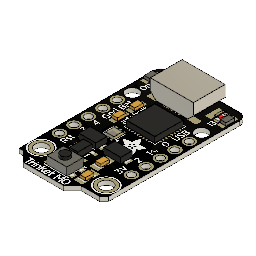
3500 Trinket M0 (Autodesk Fusion 360 design; units mm, degrees)
Autodesk Fusion 360 part; units mm, degrees
sketch "pcb" plane through (0, 0, 0) normal (0, 0, 1) x (1, 0, 0)
  arc A0 (7.62, 11.43) -> (6.35, 12.7) centre (6.35, 11.43) ccw
  line L0 (-6.858, -12.192) -> (-7.62, -12.192)
  line L1 (-7.62, -12.192) -> (-7.62, 11.43)
  line L2 (2.413, 12.319) -> (2.794, 12.7)
  line L3 (7.62, -11.684) -> (6.858, -12.446)
  line L4 (6.858, -12.446) -> (3.556, -12.446)
  line L5 (2.032, -13.97) -> (-5.08, -13.97)
  line L6 (3.556, -12.446) -> (2.032, -13.97)
  line L7 (-2.794, 12.7) -> (-2.413, 12.319)
  circle A1 centre (6.096, 6.223) radius 1.1
  line L8 (2.794, 12.7) -> (6.35, 12.7)
  arc A2 (-6.35, 12.7) -> (-7.62, 11.43) centre (-6.35, 11.43) ccw
  line L9 (-6.35, 12.7) -> (-2.794, 12.7)
  circle A3 centre (-6.096, 6.223) radius 1.1
  line L10 (-2.413, 12.319) -> (2.413, 12.319)
  line L11 (7.62, 11.43) -> (7.62, -11.684)
  line L12 (-5.08, -13.97) -> (-6.858, -12.192)
  circle A4 centre (-6.3246, 3.81) radius 0.635
  circle A5 centre (6.35, 3.81) radius 0.635
  circle A6 centre (6.35, 1.27) radius 0.635
  circle A7 centre (6.35, -1.27) radius 0.635
  circle A8 centre (6.35, -3.81) radius 0.635
  circle A9 centre (6.35, -6.35) radius 0.635
  circle A10 centre (-6.3246, 1.27) radius 0.635
  circle A11 centre (-6.3246, -1.27) radius 0.635
  circle A12 centre (-6.3246, -3.81) radius 0.635
  circle A13 centre (-6.3246, -6.35) radius 0.635
  circle A14 centre (-5.715, -10.16) radius 1.1
  circle A15 centre (5.715, -10.16) radius 1.1
  dimension "d1" = 1.27
  dimension "d2" = 1.27
  dimension "d5" = 0
  dimension "d6" = -2.54
  dimension "d9" = 0
  dimension "d10" = -2.54
  dimension "d11" = 2.2
  dimension "d12" = 2.2
  dimension "d13" = 2.2
  dimension "d14" = 2.2
  measures "d1" diameter of A4
  measures "d2" diameter of A5
  measures "d11" diameter of A14
  measures "d12" diameter of A15
  measures "d13" diameter of A1
  measures "d14" diameter of A3
extrude "Extrude1" add sketch "pcb" along normal blind 0.8 makes body 1
sketch "usb" plane through (0, 0, 0.8) normal (0, 0, 1) x (-1, 0, 0)
  circle A0 centre (-6.35, -3.81) radius 0.635
  circle A1 centre (-6.35, 6.35) radius 0.635
  circle A2 centre (5.715, 10.16) radius 1.1
  circle A3 centre (6.3246, -3.81) radius 0.635
  circle A4 centre (6.3246, 6.35) radius 0.635
  circle A5 centre (-6.096, -6.223) radius 1.1
  circle A6 centre (-6.35, -1.27) radius 0.635
  circle A7 centre (6.3246, -1.27) radius 0.635
  circle A8 centre (6.096, -6.223) radius 1.1
  circle A9 centre (6.3246, 1.27) radius 0.635
  circle A10 centre (-5.715, 10.16) radius 1.1
  circle A11 centre (-6.35, 1.27) radius 0.635
  circle A12 centre (-6.35, 3.81) radius 0.635
  circle A13 centre (6.3246, 3.81) radius 0.635
  arc A14 (-7.62, -11.43) -> (-6.35, -12.7) centre (-6.35, -11.43) ccw
  line L0 (-6.35, -12.7) -> (-2.794, -12.7)
  line L1 (-2.794, -12.7) -> (-2.413, -12.319)
  line L2 (-2.413, -12.319) -> (2.413, -12.319)
  line L3 (2.413, -12.319) -> (2.794, -12.7)
  line L4 (2.794, -12.7) -> (6.35, -12.7)
  arc A15 (6.35, -12.7) -> (7.62, -11.43) centre (6.35, -11.43) ccw
  line L5 (7.62, -11.43) -> (7.62, 12.192)
  line L6 (7.62, 12.192) -> (6.858, 12.192)
  line L7 (6.858, 12.192) -> (5.08, 13.97)
  line L8 (5.08, 13.97) -> (-2.032, 13.97)
  line L9 (-2.032, 13.97) -> (-3.556, 12.446)
  line L10 (-3.556, 12.446) -> (-6.858, 12.446)
  line L11 (-6.858, 12.446) -> (-7.62, 11.684)
  line L12 (-7.62, 11.684) -> (-7.62, -11.43)
  line L13 (3.8, -12.7) -> (-3.8, -12.7)
  line L14 (-3.8, -12.7) -> (-3.8, -7.1)
  line L15 (-3.8, -7.1) -> (3.8, -7.1)
  line L16 (3.8, -7.1) -> (3.8, -12.7)
  line L17 (3.8, -12.7) -> (-3.8, -7.1) construction
  line L18 (-3.8, -12.7) -> (3.8, -7.1) construction
  line L19 (0, -9.9) -> (0, 0) construction
  point P0 (0, -9.9)
  dimension "d17" = 7.6
  dimension "d18" = 5.6
  dimension "d19" = 9.9
  measures "d17" distance of L14.end L15.end
  measures "d18" distance of L13.end L14.end
  measures "d19" distance of L19.end L19.start
extrude "Extrude2" add sketch "usb" along normal blind 3 separate body contours L0 L1 L2 L3 L4 L13 L14 L15 L16 | L1 L2 L3 L13 makes body 2
chamfer "Chamfer1" distance 1 angle 45 2 edges at (3.8, 9.9, 0.8) (-3.8, 9.9, 0.8) on bodies 2
shell "Shell1" thickness 0.4 removed faces 1 at (-0.9333, 12.7, 2.8) on bodies 2
sketch "samd21" plane through (0, 0, 0.8) normal (0, 0, 1) x (-1, 0, 0)
  circle A0 centre (-6.35, -3.81) radius 0.635
  circle A1 centre (-6.35, 6.35) radius 0.635
  circle A2 centre (5.715, 10.16) radius 1.1
  circle A3 centre (6.3246, -3.81) radius 0.635
  circle A4 centre (6.3246, 6.35) radius 0.635
  circle A5 centre (-6.096, -6.223) radius 1.1
  circle A6 centre (-6.35, -1.27) radius 0.635
  circle A7 centre (6.3246, -1.27) radius 0.635
  circle A8 centre (6.096, -6.223) radius 1.1
  circle A9 centre (6.3246, 1.27) radius 0.635
  circle A10 centre (-5.715, 10.16) radius 1.1
  circle A11 centre (-6.35, 1.27) radius 0.635
  circle A12 centre (-6.35, 3.81) radius 0.635
  circle A13 centre (6.3246, 3.81) radius 0.635
  arc A14 (-7.62, -11.43) -> (-6.35, -12.7) centre (-6.35, -11.43) ccw
  line L0 (-6.35, -12.7) -> (-2.794, -12.7)
  line L1 (-2.794, -12.7) -> (-2.413, -12.319)
  line L2 (-2.413, -12.319) -> (2.413, -12.319)
  line L3 (2.413, -12.319) -> (2.794, -12.7)
  line L4 (2.794, -12.7) -> (6.35, -12.7)
  arc A15 (6.35, -12.7) -> (7.62, -11.43) centre (6.35, -11.43) ccw
  line L5 (7.62, -11.43) -> (7.62, 12.192)
  line L6 (7.62, 12.192) -> (6.858, 12.192)
  line L7 (6.858, 12.192) -> (5.08, 13.97)
  line L8 (5.08, 13.97) -> (-2.032, 13.97)
  line L9 (-2.032, 13.97) -> (-3.556, 12.446)
  line L10 (-3.556, 12.446) -> (-6.858, 12.446)
  line L11 (-6.858, 12.446) -> (-7.62, 11.684)
  line L12 (-7.62, 11.684) -> (-7.62, -11.43)
  line L13 (-3.5719, -0.5328) -> (1.4281, -0.5328)
  line L14 (1.4281, -0.5328) -> (1.4281, -5.5328)
  line L15 (1.4281, -5.5328) -> (-3.5719, -5.5328)
  line L16 (-3.5719, -5.5328) -> (-3.5719, -0.5328)
  line L17 (-3.5719, -0.5328) -> (1.4281, -5.5328) construction
  line L18 (1.4281, -0.5328) -> (-3.5719, -5.5328) construction
  point P0 (-1.0719, -3.0328)
  dimension "d24" = 5
  dimension "d25" = 5
  dimension "d26" = 3.0328
  dimension "d27" = 1.0719
  measures "d24" distance of L14.end L15.end
  measures "d25" distance of L13.end L14.end
  measures "d26" distance of origin P0
  measures "d27" distance of origin P0
extrude "Extrude3" add sketch "samd21" along normal blind 1 separate body contours L13 L14 L15 L16 makes body 3
sketch "LEDs" plane through (0, 0, 0.8) normal (0, 0, 1) x (-1, 0, 0)
  circle A0 centre (-6.35, -3.81) radius 0.635
  circle A1 centre (-6.35, 6.35) radius 0.635
  circle A2 centre (5.715, 10.16) radius 1.1
  circle A3 centre (6.3246, -3.81) radius 0.635
  circle A4 centre (6.3246, 6.35) radius 0.635
  circle A5 centre (-6.096, -6.223) radius 1.1
  circle A6 centre (-6.35, -1.27) radius 0.635
  circle A7 centre (6.3246, -1.27) radius 0.635
  circle A8 centre (6.096, -6.223) radius 1.1
  circle A9 centre (6.3246, 1.27) radius 0.635
  circle A10 centre (-5.715, 10.16) radius 1.1
  circle A11 centre (-6.35, 1.27) radius 0.635
  circle A12 centre (-6.35, 3.81) radius 0.635
  circle A13 centre (6.3246, 3.81) radius 0.635
  arc A14 (-7.62, -11.43) -> (-6.35, -12.7) centre (-6.35, -11.43) ccw
  line L0 (-6.35, -12.7) -> (-2.794, -12.7)
  line L1 (-2.794, -12.7) -> (-2.413, -12.319)
  line L2 (-2.413, -12.319) -> (2.413, -12.319)
  line L3 (2.413, -12.319) -> (2.794, -12.7)
  line L4 (2.794, -12.7) -> (6.35, -12.7)
  arc A15 (6.35, -12.7) -> (7.62, -11.43) centre (6.35, -11.43) ccw
  line L5 (7.62, -11.43) -> (7.62, 12.192)
  line L6 (7.62, 12.192) -> (6.858, 12.192)
  line L7 (6.858, 12.192) -> (5.08, 13.97)
  line L8 (5.08, 13.97) -> (-2.032, 13.97)
  line L9 (-2.032, 13.97) -> (-3.556, 12.446)
  line L10 (-3.556, 12.446) -> (-6.858, 12.446)
  line L11 (-6.858, 12.446) -> (-7.62, 11.684)
  line L12 (-7.62, 11.684) -> (-7.62, -11.43)
  line L13 (6.0245, -9.537) -> (5.0245, -9.537)
  line L14 (5.0245, -9.537) -> (5.0245, -11.037)
  line L15 (5.0245, -11.037) -> (6.0245, -11.037)
  line L16 (6.0245, -11.037) -> (6.0245, -9.537)
  line L17 (6.0245, -9.537) -> (5.0245, -11.037) construction
  line L18 (5.0245, -9.537) -> (6.0245, -11.037) construction
  line L19 (7.231, -9.41) -> (6.231, -9.41)
  line L20 (6.231, -9.41) -> (6.231, -10.91)
  line L21 (6.231, -10.91) -> (7.231, -10.91)
  line L22 (7.231, -10.91) -> (7.231, -9.41)
  line L23 (7.231, -9.41) -> (6.231, -10.91) construction
  line L24 (6.231, -9.41) -> (7.231, -10.91) construction
  line L25 (-5.0245, -9.537) -> (-6.0245, -9.537)
  line L26 (-6.0245, -9.537) -> (-6.0245, -11.037)
  line L27 (-6.0245, -11.037) -> (-5.0245, -11.037)
  line L28 (-5.0245, -11.037) -> (-5.0245, -9.537)
  line L29 (-5.0245, -9.537) -> (-6.0245, -11.037) construction
  line L30 (-6.0245, -9.537) -> (-5.0245, -11.037) construction
  line L31 (-6.231, -9.3846) -> (-7.231, -9.3846)
  line L32 (-7.231, -9.3846) -> (-7.231, -10.8846)
  line L33 (-7.231, -10.8846) -> (-6.231, -10.8846)
  line L34 (-6.231, -10.8846) -> (-6.231, -9.3846)
  line L35 (-6.231, -9.3846) -> (-7.231, -10.8846) construction
  line L36 (-7.231, -9.3846) -> (-6.231, -10.8846) construction
  point P0 (5.5245, -10.287)
  point P1 (6.731, -10.16)
  point P2 (-5.5245, -10.287)
  point P3 (-6.731, -10.1346)
  dimension "d30" = 1
  dimension "d31" = 1.5
  dimension "d32" = 1.5
  dimension "d33" = 1
  dimension "d34" = 6.731
  dimension "d35" = 10.16
  dimension "d36" = 10.287
  dimension "d37" = 5.5245
  dimension "d38" = 1.5
  dimension "d39" = 1
  dimension "d40" = 1
  dimension "d41" = 1.5
  dimension "d42" = 10.287
  dimension "d43" = 5.5245
  dimension "d44" = 6.731
  dimension "d45" = 10.1346
  measures "d30" distance of L14.end L15.end
  measures "d31" distance of L13.end L14.end
  measures "d32" distance of L19.end L20.end
  measures "d33" distance of L20.end L21.end
  measures "d34" distance of origin P1
  measures "d35" distance of origin P1
  measures "d36" distance of origin P0
  measures "d37" distance of origin P0
  measures "d38" distance of L25.end L26.end
  measures "d39" distance of L26.end L27.end
  measures "d40" distance of L32.end L33.end
  measures "d41" distance of L31.end L32.end
  measures "d42" distance of origin P2
  measures "d43" distance of origin P2
  measures "d44" distance of origin P3
  measures "d45" distance of origin P3
extrude "Extrude4" add sketch "LEDs" along normal blind 0.5 separate body contours L13 L14 L15 L16 | L19 L20 L21 L22 | L25 L26 L27 L28 | L31 L32 L33 L34 makes body 4 at (-6.5643, 10.41, 0.8) makes body 5 at (-5.6912, 10.037, 0.8) makes body 6 at (6.8977, 9.8846, 0.8) makes body 7 at (5.6912, 10.037, 0.8)
sketch "caps" plane through (0, 0, 0.8) normal (0, 0, 1) x (-1, 0, 0)
  circle A0 centre (-6.35, -3.81) radius 0.635
  circle A1 centre (-6.35, 6.35) radius 0.635
  circle A2 centre (5.715, 10.16) radius 1.1
  circle A3 centre (6.3246, -3.81) radius 0.635
  circle A4 centre (6.3246, 6.35) radius 0.635
  circle A5 centre (-6.096, -6.223) radius 1.1
  circle A6 centre (-6.35, -1.27) radius 0.635
  circle A7 centre (6.3246, -1.27) radius 0.635
  circle A8 centre (6.096, -6.223) radius 1.1
  circle A9 centre (6.3246, 1.27) radius 0.635
  circle A10 centre (-5.715, 10.16) radius 1.1
  circle A11 centre (-6.35, 1.27) radius 0.635
  circle A12 centre (-6.35, 3.81) radius 0.635
  circle A13 centre (6.3246, 3.81) radius 0.635
  arc A14 (-7.62, -11.43) -> (-6.35, -12.7) centre (-6.35, -11.43) ccw
  line L0 (-6.35, -12.7) -> (-2.794, -12.7)
  line L1 (-2.794, -12.7) -> (-2.413, -12.319)
  line L2 (-2.413, -12.319) -> (2.413, -12.319)
  line L3 (2.413, -12.319) -> (2.794, -12.7)
  line L4 (2.794, -12.7) -> (6.35, -12.7)
  arc A15 (6.35, -12.7) -> (7.62, -11.43) centre (6.35, -11.43) ccw
  line L5 (7.62, -11.43) -> (7.62, 12.192)
  line L6 (7.62, 12.192) -> (6.858, 12.192)
  line L7 (6.858, 12.192) -> (5.08, 13.97)
  line L8 (5.08, 13.97) -> (-2.032, 13.97)
  line L9 (-2.032, 13.97) -> (-3.556, 12.446)
  line L10 (-3.556, 12.446) -> (-6.858, 12.446)
  line L11 (-6.858, 12.446) -> (-7.62, 11.684)
  line L12 (-7.62, 11.684) -> (-7.62, -11.43)
  line L13 (3.056, -3.6315) -> (4.056, -3.6315)
  line L14 (4.056, -3.6315) -> (4.056, -5.1315)
  line L15 (4.056, -5.1315) -> (3.056, -5.1315)
  line L16 (3.056, -5.1315) -> (3.056, -3.6315)
  line L17 (3.056, -3.6315) -> (4.056, -5.1315) construction
  line L18 (4.056, -3.6315) -> (3.056, -5.1315) construction
  line L19 (3.056, -0.5835) -> (4.056, -0.5835)
  line L20 (4.056, -0.5835) -> (4.056, -2.0835)
  line L21 (4.056, -2.0835) -> (3.056, -2.0835)
  line L22 (3.056, -2.0835) -> (3.056, -0.5835)
  line L23 (3.056, -0.5835) -> (4.056, -2.0835) construction
  line L24 (4.056, -0.5835) -> (3.056, -2.0835) construction
  point P0 (3.556, -4.3815)
  point P1 (3.556, -1.3335)
  dimension "d48" = 1.5
  dimension "d49" = 1
  dimension "d50" = 3.556
  dimension "d51" = 4.3815
  dimension "d52" = 1.5
  dimension "d53" = 1
  dimension "d54" = 1.3335
  measures "d48" distance of L13.end L14.end
  measures "d49" distance of L14.end L15.end
  measures "d50" distance of origin P0
  measures "d51" distance of origin P0
  measures "d52" distance of L19.end L20.end
  measures "d53" distance of L20.end L21.end
  measures "d54" distance of origin P1
extrude "Extrude5" add sketch "caps" along normal blind 0.5 separate body contours L13 L14 L15 L16 | L19 L20 L21 L22 makes body 8 at (-3.3893, 1.0835, 0.8) makes body 9 at (-3.7227, 4.6315, 0.8)
sketch "dotstar" plane through (0, 0, 0.8) normal (0, 0, 1) x (-1, 0, 0)
  circle A0 centre (-6.35, -3.81) radius 0.635
  circle A1 centre (-6.35, 6.35) radius 0.635
  circle A2 centre (5.715, 10.16) radius 1.1
  circle A3 centre (6.3246, -3.81) radius 0.635
  circle A4 centre (6.3246, 6.35) radius 0.635
  circle A5 centre (-6.096, -6.223) radius 1.1
  circle A6 centre (-6.35, -1.27) radius 0.635
  circle A7 centre (6.3246, -1.27) radius 0.635
  circle A8 centre (6.096, -6.223) radius 1.1
  circle A9 centre (6.3246, 1.27) radius 0.635
  circle A10 centre (-5.715, 10.16) radius 1.1
  circle A11 centre (-6.35, 1.27) radius 0.635
  circle A12 centre (-6.35, 3.81) radius 0.635
  circle A13 centre (6.3246, 3.81) radius 0.635
  arc A14 (-7.62, -11.43) -> (-6.35, -12.7) centre (-6.35, -11.43) ccw
  line L0 (-6.35, -12.7) -> (-2.794, -12.7)
  line L1 (-2.794, -12.7) -> (-2.413, -12.319)
  line L2 (-2.413, -12.319) -> (2.413, -12.319)
  line L3 (2.413, -12.319) -> (2.794, -12.7)
  line L4 (2.794, -12.7) -> (6.35, -12.7)
  arc A15 (6.35, -12.7) -> (7.62, -11.43) centre (6.35, -11.43) ccw
  line L5 (7.62, -11.43) -> (7.62, 12.192)
  line L6 (7.62, 12.192) -> (6.858, 12.192)
  line L7 (6.858, 12.192) -> (5.08, 13.97)
  line L8 (5.08, 13.97) -> (-2.032, 13.97)
  line L9 (-2.032, 13.97) -> (-3.556, 12.446)
  line L10 (-3.556, 12.446) -> (-6.858, 12.446)
  line L11 (-6.858, 12.446) -> (-7.62, 11.684)
  line L12 (-7.62, 11.684) -> (-7.62, -11.43)
  line L13 (0.5037, 2.6002) -> (2.5037, 2.6002)
  line L14 (2.5037, 2.6002) -> (2.5037, 0.6002)
  line L15 (2.5037, 0.6002) -> (0.5037, 0.6002)
  line L16 (0.5037, 0.6002) -> (0.5037, 2.6002)
  line L17 (0.5037, 2.6002) -> (2.5037, 0.6002) construction
  line L18 (2.5037, 2.6002) -> (0.5037, 0.6002) construction
  point P0 (1.5037, 1.6002)
  dimension "d57" = 2
  dimension "d58" = 2
  dimension "d59" = 1.6002
  dimension "d60" = 1.5037
  measures "d57" distance of L14.end L15.end
  measures "d58" distance of L13.end L14.end
  measures "d59" distance of origin P0
  measures "d60" distance of origin P0
extrude "Extrude6" add sketch "dotstar" along normal blind 0.5 separate body contours L13 L14 L15 L16 makes body 10
sketch "reset" plane through (0, 0, 0.8) normal (0, 0, 1) x (-1, 0, 0)
  circle A0 centre (-6.35, -3.81) radius 0.635
  circle A1 centre (-6.35, 6.35) radius 0.635
  circle A2 centre (5.715, 10.16) radius 1.1
  circle A3 centre (6.3246, -3.81) radius 0.635
  circle A4 centre (6.3246, 6.35) radius 0.635
  circle A5 centre (-6.096, -6.223) radius 1.1
  circle A6 centre (-6.35, -1.27) radius 0.635
  circle A7 centre (6.3246, -1.27) radius 0.635
  circle A8 centre (6.096, -6.223) radius 1.1
  circle A9 centre (6.3246, 1.27) radius 0.635
  circle A10 centre (-5.715, 10.16) radius 1.1
  circle A11 centre (-6.35, 1.27) radius 0.635
  circle A12 centre (-6.35, 3.81) radius 0.635
  circle A13 centre (6.3246, 3.81) radius 0.635
  arc A14 (-7.62, -11.43) -> (-6.35, -12.7) centre (-6.35, -11.43) ccw
  line L0 (-6.35, -12.7) -> (-2.794, -12.7)
  line L1 (-2.794, -12.7) -> (-2.413, -12.319)
  line L2 (-2.413, -12.319) -> (2.413, -12.319)
  line L3 (2.413, -12.319) -> (2.794, -12.7)
  line L4 (2.794, -12.7) -> (6.35, -12.7)
  arc A15 (6.35, -12.7) -> (7.62, -11.43) centre (6.35, -11.43) ccw
  line L5 (7.62, -11.43) -> (7.62, 12.192)
  line L6 (7.62, 12.192) -> (6.858, 12.192)
  line L7 (6.858, 12.192) -> (5.08, 13.97)
  line L8 (5.08, 13.97) -> (-2.032, 13.97)
  line L9 (-2.032, 13.97) -> (-3.556, 12.446)
  line L10 (-3.556, 12.446) -> (-6.858, 12.446)
  line L11 (-6.858, 12.446) -> (-7.62, 11.684)
  line L12 (-7.62, 11.684) -> (-7.62, -11.43)
  line L13 (-0.861, 12.2501) -> (2.639, 12.2501)
  line L14 (2.639, 12.2501) -> (2.639, 9.3501)
  line L15 (2.639, 9.3501) -> (-0.861, 9.3501)
  line L16 (-0.861, 9.3501) -> (-0.861, 12.2501)
  line L17 (-0.861, 12.2501) -> (2.639, 9.3501) construction
  line L18 (2.639, 12.2501) -> (-0.861, 9.3501) construction
  circle A16 centre (0.889, 10.8001) radius 0.8
  point P0 (0.889, 10.8001)
  dimension "d63" = 2.9
  dimension "d64" = 3.5
  dimension "d65" = 1.6
  dimension "d66" = 0.889
  dimension "d67" = 10.8001
  measures "d63" distance of L13.end L14.end
  measures "d64" distance of L14.end L15.end
  measures "d65" diameter of A16
  measures "d66" distance of origin A16.centre
  measures "d67" distance of origin A16.centre
extrude "Extrude7" add sketch "reset" along normal blind 1.4 separate body contours L13 L14 L15 L16 | A16 makes body 11
extrude "Extrude8" add sketch "reset" along normal blind 0.5 from surface at 1.4 contours A16 bodies 11
sketch "10uF" plane through (0, 0, 0.8) normal (0, 0, 1) x (-1, 0, 0)
  circle A0 centre (-6.35, -3.81) radius 0.635
  circle A1 centre (-6.35, 6.35) radius 0.635
  circle A2 centre (5.715, 10.16) radius 1.1
  circle A3 centre (6.3246, -3.81) radius 0.635
  circle A4 centre (6.3246, 6.35) radius 0.635
  circle A5 centre (-6.096, -6.223) radius 1.1
  circle A6 centre (-6.35, -1.27) radius 0.635
  circle A7 centre (6.3246, -1.27) radius 0.635
  circle A8 centre (6.096, -6.223) radius 1.1
  circle A9 centre (6.3246, 1.27) radius 0.635
  circle A10 centre (-5.715, 10.16) radius 1.1
  circle A11 centre (-6.35, 1.27) radius 0.635
  circle A12 centre (-6.35, 3.81) radius 0.635
  circle A13 centre (6.3246, 3.81) radius 0.635
  arc A14 (-7.62, -11.43) -> (-6.35, -12.7) centre (-6.35, -11.43) ccw
  line L0 (-6.35, -12.7) -> (-2.794, -12.7)
  line L1 (-2.794, -12.7) -> (-2.413, -12.319)
  line L2 (-2.413, -12.319) -> (2.413, -12.319)
  line L3 (2.413, -12.319) -> (2.794, -12.7)
  line L4 (2.794, -12.7) -> (6.35, -12.7)
  arc A15 (6.35, -12.7) -> (7.62, -11.43) centre (6.35, -11.43) ccw
  line L5 (7.62, -11.43) -> (7.62, 12.192)
  line L6 (7.62, 12.192) -> (6.858, 12.192)
  line L7 (6.858, 12.192) -> (5.08, 13.97)
  line L8 (5.08, 13.97) -> (-2.032, 13.97)
  line L9 (-2.032, 13.97) -> (-3.556, 12.446)
  line L10 (-3.556, 12.446) -> (-6.858, 12.446)
  line L11 (-6.858, 12.446) -> (-7.62, 11.684)
  line L12 (-7.62, 11.684) -> (-7.62, -11.43)
  line L13 (-3.2305, 11.3545) -> (-2.2305, 11.3545)
  line L14 (-2.2305, 11.3545) -> (-2.2305, 9.8545)
  line L15 (-2.2305, 9.8545) -> (-3.2305, 9.8545)
  line L16 (-3.2305, 9.8545) -> (-3.2305, 11.3545)
  line L17 (-3.2305, 11.3545) -> (-2.2305, 9.8545) construction
  line L18 (-2.2305, 11.3545) -> (-3.2305, 9.8545) construction
  point P0 (-2.7305, 10.6045)
  dimension "d73" = 1
  dimension "d74" = 1.5
  dimension "d75" = 10.6045
  dimension "d76" = 2.7305
  measures "d73" distance of L14.end L15.end
  measures "d74" distance of L13.end L14.end
  measures "d75" distance of origin P0
  measures "d76" distance of origin P0
extrude "Extrude9" add sketch "10uF" along normal blind 0.5 separate body contours L13 L14 L15 L16 makes body 12
sketch "cap" plane through (0, 0, 0.8) normal (0, 0, 1) x (-1, 0, 0)
  circle A0 centre (-6.35, -3.81) radius 0.635
  circle A1 centre (-6.35, 6.35) radius 0.635
  circle A2 centre (5.715, 10.16) radius 1.1
  circle A3 centre (6.3246, -3.81) radius 0.635
  circle A4 centre (6.3246, 6.35) radius 0.635
  circle A5 centre (-6.096, -6.223) radius 1.1
  circle A6 centre (-6.35, -1.27) radius 0.635
  circle A7 centre (6.3246, -1.27) radius 0.635
  circle A8 centre (6.096, -6.223) radius 1.1
  circle A9 centre (6.3246, 1.27) radius 0.635
  circle A10 centre (-5.715, 10.16) radius 1.1
  circle A11 centre (-6.35, 1.27) radius 0.635
  circle A12 centre (-6.35, 3.81) radius 0.635
  circle A13 centre (6.3246, 3.81) radius 0.635
  arc A14 (-7.62, -11.43) -> (-6.35, -12.7) centre (-6.35, -11.43) ccw
  line L0 (-6.35, -12.7) -> (-2.794, -12.7)
  line L1 (-2.794, -12.7) -> (-2.413, -12.319)
  line L2 (-2.413, -12.319) -> (2.413, -12.319)
  line L3 (2.413, -12.319) -> (2.794, -12.7)
  line L4 (2.794, -12.7) -> (6.35, -12.7)
  arc A15 (6.35, -12.7) -> (7.62, -11.43) centre (6.35, -11.43) ccw
  line L5 (7.62, -11.43) -> (7.62, 12.192)
  line L6 (7.62, 12.192) -> (6.858, 12.192)
  line L7 (6.858, 12.192) -> (5.08, 13.97)
  line L8 (5.08, 13.97) -> (-2.032, 13.97)
  line L9 (-2.032, 13.97) -> (-3.556, 12.446)
  line L10 (-3.556, 12.446) -> (-6.858, 12.446)
  line L11 (-6.858, 12.446) -> (-7.62, 11.684)
  line L12 (-7.62, 11.684) -> (-7.62, -11.43)
  line L13 (-2.532, 7.9255) -> (-1.532, 7.9255)
  line L14 (-1.532, 7.9255) -> (-1.532, 6.4255)
  line L15 (-1.532, 6.4255) -> (-2.532, 6.4255)
  line L16 (-2.532, 6.4255) -> (-2.532, 7.9255)
  line L17 (-2.532, 7.9255) -> (-1.532, 6.4255) construction
  line L18 (-1.532, 7.9255) -> (-2.532, 6.4255) construction
  point P0 (-2.032, 7.1755)
  dimension "d79" = 1.5
  dimension "d80" = 1
  dimension "d81" = 2.032
  dimension "d82" = 7.1755
  measures "d79" distance of L13.end L14.end
  measures "d80" distance of L14.end L15.end
  measures "d81" distance of origin P0
  measures "d82" distance of origin P0
extrude "Extrude10" add sketch "cap" along normal blind 0.5 separate body contours L13 L14 L15 L16 makes body 13
sketch "AP2112K" plane through (0, 0, 0.8) normal (0, 0, 1) x (-1, 0, 0)
  circle A0 centre (-6.35, -3.81) radius 0.635
  circle A1 centre (-6.35, 6.35) radius 0.635
  circle A2 centre (5.715, 10.16) radius 1.1
  circle A3 centre (6.3246, -3.81) radius 0.635
  circle A4 centre (6.3246, 6.35) radius 0.635
  circle A5 centre (-6.096, -6.223) radius 1.1
  circle A6 centre (-6.35, -1.27) radius 0.635
  circle A7 centre (6.3246, -1.27) radius 0.635
  circle A8 centre (6.096, -6.223) radius 1.1
  circle A9 centre (6.3246, 1.27) radius 0.635
  circle A10 centre (-5.715, 10.16) radius 1.1
  circle A11 centre (-6.35, 1.27) radius 0.635
  circle A12 centre (-6.35, 3.81) radius 0.635
  circle A13 centre (6.3246, 3.81) radius 0.635
  arc A14 (-7.62, -11.43) -> (-6.35, -12.7) centre (-6.35, -11.43) ccw
  line L0 (-6.35, -12.7) -> (-2.794, -12.7)
  line L1 (-2.794, -12.7) -> (-2.413, -12.319)
  line L2 (-2.413, -12.319) -> (2.413, -12.319)
  line L3 (2.413, -12.319) -> (2.794, -12.7)
  line L4 (2.794, -12.7) -> (6.35, -12.7)
  arc A15 (6.35, -12.7) -> (7.62, -11.43) centre (6.35, -11.43) ccw
  line L5 (7.62, -11.43) -> (7.62, 12.192)
  line L6 (7.62, 12.192) -> (6.858, 12.192)
  line L7 (6.858, 12.192) -> (5.08, 13.97)
  line L8 (5.08, 13.97) -> (-2.032, 13.97)
  line L9 (-2.032, 13.97) -> (-3.556, 12.446)
  line L10 (-3.556, 12.446) -> (-6.858, 12.446)
  line L11 (-6.858, 12.446) -> (-7.62, 11.684)
  line L12 (-7.62, 11.684) -> (-7.62, -11.43)
  line L13 (0.8375, 8.616) -> (2.3375, 8.616)
  line L14 (2.3375, 8.616) -> (2.3375, 6.116)
  line L15 (2.3375, 6.116) -> (0.8375, 6.116)
  line L16 (0.8375, 6.116) -> (0.8375, 8.616)
  line L17 (0.8375, 8.616) -> (2.3375, 6.116) construction
  line L18 (2.3375, 8.616) -> (0.8375, 6.116) construction
  point P0 (1.5875, 7.366)
  dimension "d85" = 1.5
  dimension "d86" = 2.5
  dimension "d87" = 7.366
  dimension "d88" = 1.5875
  measures "d85" distance of L14.end L15.end
  measures "d86" distance of L13.end L14.end
  measures "d87" distance of origin P0
  measures "d88" distance of origin P0
extrude "Extrude11" add sketch "AP2112K" along normal blind 1 separate body contours L13 L14 L15 L16 makes body 14
sketch "SOD-123FL" plane through (0, 0, 0.8) normal (0, 0, 1) x (-1, 0, 0)
  circle A0 centre (-6.35, -3.81) radius 0.635
  circle A1 centre (-6.35, 6.35) radius 0.635
  circle A2 centre (5.715, 10.16) radius 1.1
  circle A3 centre (6.3246, -3.81) radius 0.635
  circle A4 centre (6.3246, 6.35) radius 0.635
  circle A5 centre (-6.096, -6.223) radius 1.1
  circle A6 centre (-6.35, -1.27) radius 0.635
  circle A7 centre (6.3246, -1.27) radius 0.635
  circle A8 centre (6.096, -6.223) radius 1.1
  circle A9 centre (6.3246, 1.27) radius 0.635
  circle A10 centre (-5.715, 10.16) radius 1.1
  circle A11 centre (-6.35, 1.27) radius 0.635
  circle A12 centre (-6.35, 3.81) radius 0.635
  circle A13 centre (6.3246, 3.81) radius 0.635
  arc A14 (-7.62, -11.43) -> (-6.35, -12.7) centre (-6.35, -11.43) ccw
  line L0 (-6.35, -12.7) -> (-2.794, -12.7)
  line L1 (-2.794, -12.7) -> (-2.413, -12.319)
  line L2 (-2.413, -12.319) -> (2.413, -12.319)
  line L3 (2.413, -12.319) -> (2.794, -12.7)
  line L4 (2.794, -12.7) -> (6.35, -12.7)
  arc A15 (6.35, -12.7) -> (7.62, -11.43) centre (6.35, -11.43) ccw
  line L5 (7.62, -11.43) -> (7.62, 12.192)
  line L6 (7.62, 12.192) -> (6.858, 12.192)
  line L7 (6.858, 12.192) -> (5.08, 13.97)
  line L8 (5.08, 13.97) -> (-2.032, 13.97)
  line L9 (-2.032, 13.97) -> (-3.556, 12.446)
  line L10 (-3.556, 12.446) -> (-6.858, 12.446)
  line L11 (-6.858, 12.446) -> (-7.62, 11.684)
  line L12 (-7.62, 11.684) -> (-7.62, -11.43)
  line L13 (0.659, 5.6355) -> (3.659, 5.6355)
  line L14 (3.659, 5.6355) -> (3.659, 3.6355)
  line L15 (3.659, 3.6355) -> (0.659, 3.6355)
  line L16 (0.659, 3.6355) -> (0.659, 5.6355)
  line L17 (0.659, 5.6355) -> (3.659, 3.6355) construction
  line L18 (3.659, 5.6355) -> (0.659, 3.6355) construction
  point P0 (2.159, 4.6355)
  dimension "d91" = 2
  dimension "d92" = 3
  dimension "d93" = 4.6355
  dimension "d94" = 2.159
  measures "d91" distance of L13.end L14.end
  measures "d92" distance of L14.end L15.end
  measures "d93" distance of origin P0
  measures "d94" distance of origin P0
extrude "Extrude12" add sketch "SOD-123FL" along normal blind 1 separate body contours L13 L14 L15 L16 makes body 15
sketch "Sketch12" plane through (0, 0, 0.8) normal (0, 0, 1) x (-1, 0, 0)
  circle A0 centre (-6.35, -3.81) radius 0.635
  circle A1 centre (-6.35, 6.35) radius 0.635
  circle A2 centre (5.715, 10.16) radius 1.1
  circle A3 centre (6.3246, -3.81) radius 0.635
  circle A4 centre (6.3246, 6.35) radius 0.635
  circle A5 centre (-6.096, -6.223) radius 1.1
  circle A6 centre (-6.35, -1.27) radius 0.635
  circle A7 centre (6.3246, -1.27) radius 0.635
  circle A8 centre (6.096, -6.223) radius 1.1
  circle A9 centre (6.3246, 1.27) radius 0.635
  circle A10 centre (-5.715, 10.16) radius 1.1
  circle A11 centre (-6.35, 1.27) radius 0.635
  circle A12 centre (-6.35, 3.81) radius 0.635
  circle A13 centre (6.3246, 3.81) radius 0.635
  arc A14 (-7.62, -11.43) -> (-6.35, -12.7) centre (-6.35, -11.43) ccw
  line L0 (-6.35, -12.7) -> (-2.794, -12.7)
  line L1 (-2.794, -12.7) -> (-2.413, -12.319)
  line L2 (-2.413, -12.319) -> (2.413, -12.319)
  line L3 (2.413, -12.319) -> (2.794, -12.7)
  line L4 (2.794, -12.7) -> (6.35, -12.7)
  arc A15 (6.35, -12.7) -> (7.62, -11.43) centre (6.35, -11.43) ccw
  line L5 (7.62, -11.43) -> (7.62, 12.192)
  line L6 (7.62, 12.192) -> (6.858, 12.192)
  line L7 (6.858, 12.192) -> (5.08, 13.97)
  line L8 (5.08, 13.97) -> (-2.032, 13.97)
  line L9 (-2.032, 13.97) -> (-3.556, 12.446)
  line L10 (-3.556, 12.446) -> (-6.858, 12.446)
  line L11 (-6.858, 12.446) -> (-7.62, 11.684)
  line L12 (-7.62, 11.684) -> (-7.62, -11.43)
  line L13 (-3.7352, 5.6355) -> (-0.7352, 5.6355)
  line L14 (-0.7352, 5.6355) -> (-0.7352, 3.6355)
  line L15 (-0.7352, 3.6355) -> (-3.7352, 3.6355)
  line L16 (-3.7352, 3.6355) -> (-3.7352, 5.6355)
  line L17 (-3.7352, 5.6355) -> (-0.7352, 3.6355) construction
  line L18 (-0.7352, 5.6355) -> (-3.7352, 3.6355) construction
  point P0 (-2.2352, 4.6355)
  dimension "d97" = 2
  dimension "d98" = 3
  dimension "d99" = 2.2352
  dimension "d100" = 4.6355
  measures "d97" distance of L13.end L14.end
  measures "d98" distance of L14.end L15.end
  measures "d99" distance of origin P0
  measures "d100" distance of origin P0
extrude "Extrude13" add sketch "Sketch12" along normal blind 1 separate body contours L13 L14 L15 L16 makes body 16
equation "d19 = 12.7 mm - 2.8 mm"
named bodies: "pcb", "usb", "samd21", "r1", "led on", "r2", "led red", "cap 1", "cap 2", "dotstar", "reset", "cap 3", "cap 4", "AP2112K", "SOD-123FL"
